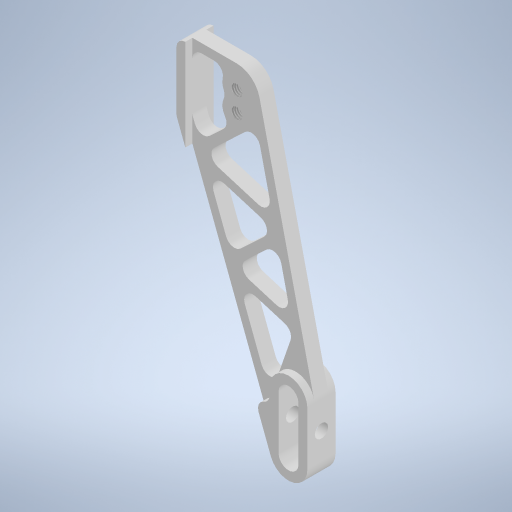
# Autodesk Inventor part: VerticalSlideMiddleTop2.2
Saved by Autodesk Inventor 2023 (Build 270158000, 158)
## iProperties
Created: 2022-10-14
Part Number: VerticalSlideMiddleTop2.2
Material: Generic
Document SubType Name: Modeling
Designer: deli
Density: 1 g/cm^3
Appearance: Default
Mass: 2.31146 g
Surface Area: 29.6295 cm^2
Volume: 2.31146 cm^3
Author: deli
Autodesk Inventor part; units mm, degrees
ref_plane "YZ Plane" through (0, 0, 0) normal (1, 0, 0) x (0, 1, 0)
ref_plane "XZ Plane" through (0, 0, 0) normal (0, 1, 0) x (-1, 0, 0)
ref_plane "XY Plane" through (0, 0, 0) normal (0, 0, 1) x (1, 0, 0)
sketch "Sketch1" plane through (0, 0, 0) normal (0, 0, 1) x (1, 0, 0)
  line L0 (-75.1619, -122.5247) -> (-75.1619, -135.5247)
  line L1 (-75.0311, -136.2362) -> (-53.8839, -191.7867)
  circle A0 centre (-63.1619, -130.2747) radius 1.25
  circle A1 centre (-63.1619, -125.7747) radius 1.25
  arc A2 (-52.1619, -190.2747) -> (-47.6619, -190.2747) centre (-49.9119, -190.2747) ccw
  arc A3 (-47.6619, -178.2747) -> (-52.1619, -178.2747) centre (-49.9119, -178.2747) ccw
  line L2 (-47.6619, -178.2747) -> (-47.6619, -190.2747)
  line L3 (-52.1619, -178.2747) -> (-52.1619, -190.2747)
  line L4 (-45.6619, -178.2747) -> (-45.6619, -190.2747)
  arc A4 (-53.8839, -191.7867) -> (-45.6619, -190.2747) centre (-49.9119, -190.2747) ccw
  arc A5 (-45.6619, -178.2747) -> (-45.7727, -177.3109) centre (-49.9119, -178.2747) ccw
  line L5 (-45.7727, -177.3109) -> (-58.0487, -124.5842)
  line L6 (-73.1619, -120.5247) -> (-63.1619, -120.5247)
  arc A6 (-58.0487, -124.5842) -> (-63.1619, -120.5247) centre (-63.1619, -125.7747) ccw
  arc A7 (-73.1619, -120.5247) -> (-75.1619, -122.5247) centre (-73.1619, -122.5247) ccw
  arc A8 (-75.1619, -135.5247) -> (-75.0311, -136.2362) centre (-73.1619, -135.5247) ccw
  line L7 (-52.1619, -182.7747) -> (-56.1619, -182.7747)
  line L8 (-56.1619, -182.7747) -> (-56.1619, -185.7747)
  line L9 (-56.1619, -185.7747) -> (-52.1619, -185.7747)
  point P0 (0, 0)
  dimension "d2" = 2.5
  dimension "d11" = 2
  dimension "d22" = 12
  dimension "d46" = 2
  dimension "d47" = 4.5
  dimension "d84" = 4
  dimension "d86" = 12
  dimension "d87" = 12
  dimension "d88" = 23
  dimension "d90" = 4
  dimension "d91" = 3
  dimension "d92" = 4.5
  dimension "d94" = 15
  dimension "d96" = 2
  dimension "d147" = 60
  constraints: 20 end point, 16 point on circle, 13 tangent, 9 centre point, 4 equal radius, 4 point on line, 3 perpendicular, 2 coincident, 2 vertical, 1 concentric, 1 horizontal, 1 parallel
  measures "d2" diameter of A0
  measures "d22" distance of A2.centre A3.centre
  measures "d46" radial gap between concentric circles of A4 A2
  measures "d47" distance between parallel lines of L2 L3
  measures "d84" distance edge to line of A1 L6
  measures "d86" distance from line of A1.centre L0
  measures "d87" distance from line of A0.centre L0
  measures "d88" distance between parallel lines of L3 L0
  measures "d90" distance of L7.start L7.end
  measures "d91" distance of L7.end L8.end
  measures "d92" distance from line of L3.start L7
  measures "d94" distance from line of L6 L0.end
  measures "d96" radius of A7
  measures "d147" vertical distance of A2.centre A0.centre
extrude "Extrusion1" add sketch "Sketch1" along normal blind 6.35 contours A7 L6 A6 L5 A5 L4 A4 L1 A8 L0 | L9 L8 L7 L3
thread "Thread2" size "M3x0.5" class "6H" standard "ANSI Metric M Profile" full length
thread "Thread6" size "M3x0.5" class "6H" standard "ANSI Metric M Profile" full length
sketch "Sketch8" plane through (-52.1619, -190.2747, 0) normal (1, 0, 0) x (0, 0, -1)
  line L0 (0, 0) -> (0, 12) construction
  line L1 (0, 12) -> (-6.35, 12) construction
  line L2 (-6.35, 0) -> (-6.35, 12) construction
  line L3 (0, 0) -> (-6.35, 0) construction
  line L4 (0, 0) -> (-6.35, 0) construction
  line L5 (-6.35, 12) -> (0, 0) construction
  line L6 (-6.35, 0) -> (0, 12) construction
  circle A0 centre (-3.175, 6) radius 1.5
  point P0 (0, 190.2747)
  dimension "d97" = 3
  constraints: 4 end point, 1 centre point, 1 midpoint
  measures "d97" diameter of A0
extrude "Extrusion7" cut sketch "Sketch8" along normal blind 10 and the other way blind 4
sketch "Sketch12" plane through (0, 0, 6.35) normal (0, 0, 1) x (1, 0, 0)
  line L0 (-75.1619, -122.5247) -> (-75.1619, -135.5247) projected
  arc A0 (-75.1619, -135.5247) -> (-75.0311, -136.2362) centre (-73.1619, -135.5247) ccw projected
  line L1 (-75.0311, -136.2362) -> (-53.8839, -191.7867) projected
  arc A1 (-53.8839, -191.7867) -> (-45.6619, -190.2747) centre (-49.9119, -190.2747) ccw projected
  line L2 (-45.6619, -190.2747) -> (-45.6619, -178.2747) projected
  arc A2 (-45.6619, -178.2747) -> (-45.7727, -177.3109) centre (-49.9119, -178.2747) ccw projected
  line L3 (-45.7727, -177.3109) -> (-58.0487, -124.5842) projected
  arc A3 (-58.0487, -124.5842) -> (-63.1619, -120.5247) centre (-63.1619, -125.7747) ccw projected
  line L4 (-63.1619, -120.5247) -> (-73.1619, -120.5247) projected
  arc A4 (-73.1619, -120.5247) -> (-75.1619, -122.5247) centre (-73.1619, -122.5247) ccw projected
  circle A5 centre (-63.1619, -130.2747) radius 1.25 projected
  circle A6 centre (-63.1619, -125.7747) radius 1.25 projected
  line L5 (-47.6619, -178.2747) -> (-47.6619, -190.2747) projected
  arc A7 (-52.1619, -190.2747) -> (-47.6619, -190.2747) centre (-49.9119, -190.2747) ccw projected
  line L6 (-52.1619, -190.2747) -> (-52.1619, -178.2747) projected
  arc A8 (-47.6619, -178.2747) -> (-52.1619, -178.2747) centre (-49.9119, -178.2747) ccw projected
  line L7 (-73.1619, -135.5247) -> (-73.1619, -122.5247)
  line L8 (-73.1619, -122.5247) -> (-63.1619, -122.5247)
  line L9 (-59.9966, -125.0377) -> (-48.5382, -174.2528)
  line L10 (-54.1619, -185.4348) -> (-73.1619, -135.5247)
  line L11 (-54.1619, -178.2747) -> (-54.1619, -185.4348)
  arc A9 (-65.5072, -128.0247) -> (-60.8167, -128.0247) centre (-63.1619, -130.2747) ccw
  arc A10 (-63.1619, -122.5247) -> (-65.5072, -128.0247) centre (-63.1619, -125.7747) ccw
  arc A11 (-60.8167, -128.0247) -> (-59.9966, -125.0377) centre (-63.1619, -125.7747) ccw
  arc A12 (-48.5382, -174.2528) -> (-54.1619, -178.2747) centre (-49.9119, -178.2747) ccw
  line L12 (-58.7109, -130.56) -> (-70.759, -141.8369)
  line L13 (-54.9688, -146.6324) -> (-70.759, -141.8369)
  line L14 (-71.5278, -139.8172) -> (-64.498, -133.2373)
  line L15 (-55.5553, -181.7747) -> (-52.1619, -181.7747)
  line L16 (-52.1619, -190.2747) -> (-52.1619, -178.2747) projected
  line L17 (-69.8592, -144.2004) -> (-54.4452, -148.8817)
  line L18 (-64.4959, -158.2891) -> (-54.4452, -148.8817)
  line L19 (-63.727, -160.3088) -> (-53.9215, -151.1309)
  line L20 (-63.727, -160.3088) -> (-50.876, -164.2117)
  line L21 (-55.5819, -181.7049) -> (-50.3523, -166.4609)
  line L22 (-62.8273, -162.6723) -> (-50.3523, -166.4609)
  point P0 (0, 0)
  point P1 (-54.1619, -181.7747)
  point P2 (-60.941, -132.6474)
  dimension "d156" = 2
  dimension "d159" = 2
  dimension "d161" = 2
  dimension "d162" = 2
  dimension "d163" = 2
  dimension "d164" = 2
  dimension "d165" = 2
  dimension "d166" = 2
  dimension "d167" = 60
  dimension "d168" = 60
  dimension "d172" = 2
  dimension "d173" = 3.5
  dimension "d175" = 2
  dimension "d177" = 2
  dimension "d178" = 2
  constraints: 29 end point, 9 point on circle, 7 point on line, 6 parallel, 4 centre point, 2 tangent, 1 perpendicular, 12 other
  measures "d156" distance between parallel lines of L0 L7
  measures "d159" radial gap between concentric circles of A5 A9
  measures "d161" radial gap between concentric circles of A10 A6
  measures "d162" radial gap between concentric circles of A11 A6
  measures "d163" distance between parallel lines of L3 L9
  measures "d164" radial gap between concentric circles of A12 A8
  measures "d165" distance between parallel lines of L6 L11
  measures "d167" angle of L9 L12
  measures "d168" angle of L13 L12
  measures "d172" distance between parallel lines of L12 L14
  measures "d173" distance from line of A2.centre L15
  measures "d175" distance between parallel lines of L13 L17
  measures "d177" distance between parallel lines of L19 L18
  measures "d178" distance between parallel lines of L20 L22
extrude "Extrusion10" cut sketch "Sketch12" against normal blind 10 contours L7 L8 A10 A9 L14 L10 | L12 L9 L13 | L17 L18 L10 | L19 L9 L20 | L22 L21 L10
fillet "Fillet6" radius 2 18 edges at (-73.1619, -122.5247, 3.175) (-63.1619, -122.5247, 3.175) (-65.5072, -128.0247, 3.175) (-64.498, -133.2373, 3.175) (-71.5278, -139.8172, 3.175) (-73.1619, -135.5247, 3.175) (-70.759, -141.8369, 3.175) (-58.7109, -130.56, 3.175) (-54.9688, -146.6324, 3.175) (-69.8592, -144.2004, 3.175) (-64.4959, -158.2891, 3.175) (-54.4452, -148.8817, 3.175) (-63.727, -160.3088, 3.175) (-53.9215, -151.1309, 3.175) (-50.876, -164.2117, 3.175) (-50.3523, -166.4609, 3.175) (-62.8273, -162.6723, 3.175) (-55.5819, -181.7049, 3.175)
sketch "Sketch13" plane through (0, 0, 6.35) normal (0, 0, 1) x (1, 0, 0)
  line L0 (-73.1619, -116.2964) -> (-54.1555, -116.2964)
  line L1 (-54.1619, -181.7747) -> (-73.1619, -181.7747)
  line L2 (-73.1619, -181.7747) -> (-73.1619, -116.2964)
  line L3 (-75.1619, -122.5247) -> (-75.1619, -135.5247) projected
  arc A0 (-47.6619, -178.2747) -> (-52.1619, -178.2747) centre (-49.9119, -178.2747) ccw projected
  line L4 (-52.1619, -190.2747) -> (-52.1619, -178.2747) projected
  line L5 (-56.7677, -143.7571) -> (-60.2863, -148.1457) projected
  line L6 (-45.7727, -177.3109) -> (-58.0487, -124.5842) projected
  line L7 (-54.1619, -190.2747) -> (-54.1619, -178.2747)
  arc A1 (-45.6619, -178.2747) -> (-54.1619, -178.2747) centre (-49.9119, -178.2747) ccw
  line L8 (-58.0487, -124.5842) -> (-54.1555, -116.2964)
  point P0 (0, 0)
  point P1 (-45.7727, -177.3109)
  dimension "d134" = 2
  dimension "d135" = 3.5
  dimension "d155" = 2
  constraints: 10 end point, 2 point on circle, 1 centre point, 1 horizontal, 1 parallel, 1 other
  measures "d134" distance between parallel lines of L3 L2
  measures "d135" distance from line of A0.centre L1
  measures "d155" distance between parallel lines of L4 L7
extrude "Extrusion11" cut sketch "Sketch13" against normal blind 1.5875
sketch "Sketch14" plane through (0, 0, 0) normal (0, 0, -1) x (-1, 0, 0)
  circle A0 centre (63.1619, -130.2747) radius 1.25 projected
  circle A1 centre (63.1619, -125.7747) radius 1.25 projected
  line L0 (73.1619, -120.5247) -> (63.1619, -120.5247) projected
  line L1 (73.1619, -124.5247) -> (73.1619, -120.5247) projected
  line L2 (57.6953, -181.7747) -> (73.1619, -141.1462) projected
  line L3 (54.1619, -181.7747) -> (57.6953, -181.7747) projected
  line L4 (58.0487, -124.5842) -> (45.7727, -177.3109) projected
  arc A2 (63.1619, -120.5247) -> (58.0487, -124.5842) centre (63.1619, -125.7747) ccw projected
  line L5 (68.261, -122.5247) -> (71.1619, -122.5247) projected
  arc A3 (66.0983, -127.1675) -> (66.3185, -125.0009) centre (63.1619, -125.7747) ccw projected
  arc A4 (65.8277, -132.1338) -> (66.0983, -128.8818) centre (63.1619, -130.2747) ccw projected
  line L6 (73.1619, -141.1462) -> (73.1619, -135.1569) projected
  arc A5 (73.0311, -135.8684) -> (73.1619, -135.1569) centre (71.1619, -135.1569) ccw projected
  arc A6 (73.1619, -124.5247) -> (71.1619, -122.5247) centre (71.1619, -124.5247) ccw projected
  arc A7 (68.261, -122.5247) -> (66.3185, -125.0009) centre (68.261, -124.5247) ccw projected
  arc A8 (66.0983, -127.1675) -> (66.0983, -128.8818) centre (67.9054, -128.0247) ccw projected
  line L7 (61.3769, -166.4821) -> (57.5488, -176.5381) projected
  line L8 (55.7544, -143.2586) -> (57.9254, -133.9339) projected
  line L9 (57.7598, -147.875) -> (65.9585, -145.385) projected
  line L10 (62.3202, -156.2527) -> (56.9743, -151.2489) projected
  arc A9 (55.7544, -143.2586) -> (58.2834, -145.6258) centre (57.7023, -143.7121) ccw projected
  line L11 (67.4444, -142.8436) -> (58.2834, -145.6258) projected
  arc A10 (67.4444, -142.8436) -> (68.2299, -139.4697) centre (66.8632, -140.9299) ccw projected
  line L12 (61.24, -132.9272) -> (68.2299, -139.4697) projected
  arc A11 (61.24, -132.9272) -> (57.9254, -133.9339) centre (59.8733, -134.3874) ccw projected
  line L13 (54.1619, -178.2747) -> (54.1619, -181.7747) projected
  arc A12 (54.1619, -178.2747) -> (45.7727, -177.3109) centre (49.9119, -178.2747) ccw projected
  line L14 (53.7879, -176.4755) -> (51.0248, -168.4213) projected
  line L15 (68.4089, -148.0103) -> (65.5561, -155.5041) projected
  line L16 (52.3354, -165.8587) -> (58.9266, -163.8569) projected
  arc A13 (65.8277, -132.1338) -> (66.1014, -134.7381) centre (67.4681, -133.2779) ccw projected
  line L17 (69.3522, -137.7808) -> (66.1014, -134.7381) projected
  arc A14 (69.3522, -137.7808) -> (72.5881, -137.0322) centre (70.7189, -136.3206) ccw projected
  line L18 (73.0311, -135.8684) -> (72.5881, -137.0322) projected
  arc A15 (62.3202, -156.2527) -> (65.5561, -155.5041) centre (63.687, -154.7925) ccw projected
  arc A16 (68.4089, -148.0103) -> (65.9585, -145.385) centre (66.5397, -147.2987) ccw projected
  arc A17 (57.7598, -147.875) -> (56.9743, -151.2489) centre (58.341, -149.7887) ccw projected
  arc A18 (53.7879, -176.4755) -> (57.5488, -176.5381) centre (55.6796, -175.8265) ccw projected
  arc A19 (61.3769, -166.4821) -> (58.9266, -163.8569) centre (59.5078, -165.7706) ccw projected
  arc A20 (52.3354, -165.8587) -> (51.0248, -168.4213) centre (52.9166, -167.7724) ccw projected
  point P0 (0, 0)
extrude "Extrusion12" cut sketch "Sketch14" against normal blind 1.5875
fillet "Fillet11" radius 2 3 edges at (-57.6953, -181.7747, 5.5562) (-57.6953, -181.7747, 0.7937) (-54.1619, -181.7747, 5.5562)
equation "\"d22\" = d17"
equation "\"d17\" = 12"
body "Solid1"
